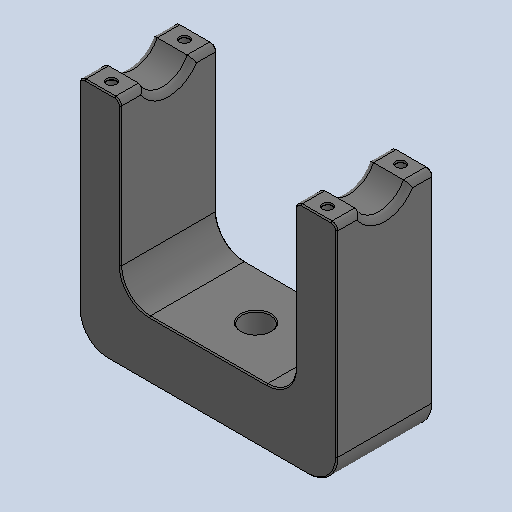
# Autodesk Inventor part: pld-support
Saved by Autodesk Inventor 2026 (Build 300175050, 175E)
## iProperties
Created: 2025-11-13
Part Number: pld-support
Material: ABS Plastic
Document SubType Name: Modeling
Designer: kuzmin
Density: 1.06 g/cm^3
Appearance: Gray
Author: kuzmin
Autodesk Inventor part; units mm, degrees
ref_plane "YZ Plane" through (0, 0, 0) normal (1, 0, 0) x (0, 1, 0)
ref_plane "XZ Plane" through (0, 0, 0) normal (0, 1, 0) x (-1, 0, 0)
ref_plane "XY Plane" through (0, 0, 0) normal (0, 0, 1) x (1, 0, 0)
sketch "Sketch1" plane through (0, 0, 0) normal (0, 0, 1) x (1, 0, 0)
  line L0 (-67, 120) -> (67, 120)
  line L1 (67, 120) -> (67, 0)
  line L2 (67, 0) -> (-67, 0)
  line L3 (-67, 0) -> (-67, 120)
  line L4 (-45.5, 120) -> (45.5, 120)
  line L5 (45.5, 120) -> (45.5, 30)
  line L6 (45.5, 30) -> (-45.5, 30)
  line L7 (-45.5, 30) -> (-45.5, 120)
  point P0 (0, 0)
  point P1 (0, 0)
  point P2 (0, 30)
  dimension "d0" = 134
  dimension "d1" = 120
  dimension "d2" = 91
  dimension "d3" = 90
  constraints: 16 end point, 4 parallel, 2 horizontal, 2 midpoint, 2 perpendicular, 1 coincident, 1 point on line, 1 vertical alignment
  measures "d0" distance of L1.end L2.end
  measures "d1" distance of L0.end L1.end
  measures "d2" distance of L5.end L6.end
  measures "d3" distance of L4.end L5.end
extrude "Extrusion1" add sketch "Sketch1" along normal mid plane 50 contours L0 L7 L6 L5 L1 L2 L3
sketch "Sketch2" plane through (-45.5, 30, -25) normal (0, 1, 0) x (1, 0, 0)
  point P0 (45.5, -25)
  point P1 (45.5, -25)
  constraints: 1 coincident
hole "Hole1" at (0, 30, 0) direction (0, -1, 0) diameter 9 end through all counterbore diameter 15 counterbore depth 15
sketch "Sketch3" plane through (67, 0, 25) normal (1, 0, 0) x (0, 0, -1)
  line L0 (50, 120) -> (0, 120) projected
  circle A0 centre (25, 126) radius 14
  point P0 (25, 0)
  point P1 (12.3509, 120)
  point P2 (37.6491, 120)
  dimension "d16" = 28
  dimension "d17" = 6
  constraints: 1 centre point
  measures "d16" diameter of A0
  measures "d17" distance from line of L0 A0.centre
extrude "Extrusion2" cut sketch "Sketch3" along normal through all both and the other way through all contours A0 L0 picked at (25, 117.3333)
fillet "Fillet1" radius 15 4 edges at (67, 0, 0) (-67, 0, 0) (-45.5, 30, 0) (45.5, 30, 0)
fillet "Fillet2" radius 3 12 edges at (-45.5, 120, -18.8246) (-67, 120, -18.8246) (-67, 120, 18.8246) (-45.5, 120, 18.8246) (45.5, 120, -18.8246) (67, 120, -18.8246) (67, 120, 18.8246) (45.5, 120, 18.8246) (45.5, 112, 0) (67, 112, 0) (-45.5, 112, 0) (-67, 112, 0)
chamfer "Chamfer1" distance 0.6 angle 45 28 edges at (-45.5, 81, 25) (-46.3787, 119.1213, 25) (-56.25, 120, 25) (-66.1213, 119.1213, 25) (-67, 66, 25) (-62.6066, 4.3934, 25) (0, 0, 25) (62.6066, 4.3934, 25) (67, 66, 25) (66.1213, 119.1213, 25) (56.25, 120, 25) (46.3787, 119.1213, 25) (45.5, 81, 25) (0, 30, 25) (67, 66, -25) (62.6066, 4.3934, -25) (0, 0, -25) (-62.6066, 4.3934, -25) (-67, 66, -25) (-66.1213, 119.1213, -25) (-56.25, 120, -25) (-46.3787, 119.1213, -25) (-45.5, 81, -25) (0, 30, -25) (45.5, 81, -25) (46.3787, 119.1213, -25) (56.25, 120, -25) (66.1213, 119.1213, -25)
sketch "Sketch4" plane through (48.5, 120, -12.6491) normal (0, 1, 0) x (1, 0, 0)
  line L0 (7.75, -31.6491) -> (7.75, 6.3509) construction
  line L1 (15.5, -37.0491) -> (0, -37.0491) projected
  point P0 (-48.5, -12.6491)
  point P1 (7.75, -37.0491)
  point P2 (7.75, -12.6491)
  dimension "d30" = 38
  constraints: 2 coincident, 2 end point, 2 midpoint, 1 horizontal alignment, 1 vertical, 1 vertical alignment
  measures "d30" distance of L0.start L0.end
hole "Hole2" at (56.25, 120, -19) at (56.25, 120, 19) direction (0, -1, 0) diameter 4.8 depth 10 tip angle 118 counterbore diameter 5.2 counterbore depth 1
mirror "Mirror1" about plane through (0, 0, 0) normal (1, 0, 0) of "Hole2"
chamfer "Chamfer2" distance 0.5 angle 45 4 edges at (0, 30, -7.5) (0, 0, -4.5) (0, 15, -4.5) (0, 15, -7.5)
equation "\"d0\" = width"
equation "\"d1\" = hight"
equation "\"d2\" = gap"
equation "\"d3\" = verticalgap"
equation "\"width\" = 134"
equation "\"hight\" = 120"
equation "\"gap\" = 91"
equation "\"verticalgap\" = 90"
body "Solid1"
